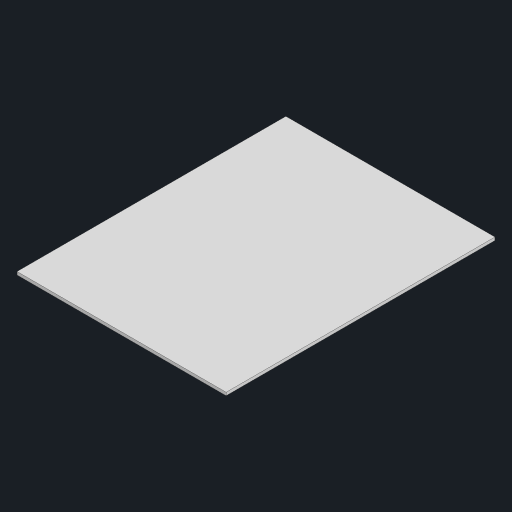
# Autodesk Inventor part: base plate
Saved by Autodesk Inventor 2024 (Build 280153000, 153)
## iProperties
Created: 2023-11-07
Part Number: base plate
Material: Generic
Document SubType Name: Modeling
Designer: 91840
Density: 1 g/cm^3
Appearance: Default
Author: 91840
Autodesk Inventor part; units mm, degrees
ref_plane "YZ Plane" through (0, 0, 0) normal (1, 0, 0) x (0, 1, 0)
ref_plane "XZ Plane" through (0, 0, 0) normal (0, 1, 0) x (-1, 0, 0)
ref_plane "XY Plane" through (0, 0, 0) normal (0, 0, 1) x (1, 0, 0)
sketch "Sketch1" plane through (0, 0, 0) normal (0, 1, 0) x (-1, 0, 0)
  line L0 (323, 12) -> (-27, 12)
  line L1 (-27, 12) -> (-27, -438)
  line L2 (-27, -438) -> (323, -438)
  line L3 (323, -438) -> (323, 12)
  point P0 (0, 0)
  dimension "d0" = 350
  dimension "d1" = 450
  dimension "d4" = 450
  constraints: 8 end point, 2 parallel, 1 horizontal, 1 perpendicular
  measures "d0" distance of L2.end L1.end
  measures "d1" distance of L1.end L0.end
  measures "d4" distance of L2.end L0.start
extrude "Extrusion1" add sketch "Sketch1" along normal blind 5
body "Solid1"
